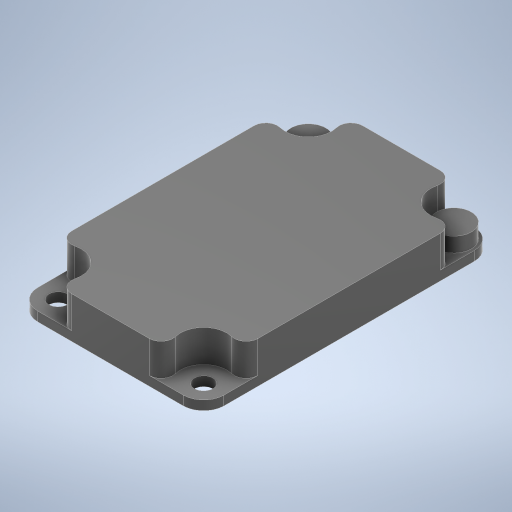
# Autodesk Inventor part: SEN0539-EN
Saved by Autodesk Inventor 2024.2 (Build 282272000, 272)
## iProperties
Created: 2024-02-11
Part Number: SEN0539-EN
Material: CFRP
Document SubType Name: Modeling
Designer: Masato Kubotera
Appearance: Smooth - Black
Surface Area: 10.415 cm^2
Volume: 0.704292 cm^3
Vendor: DFROBOT
Catalog Web Link: https://www.dfrobot.com/product-2665.html
Author: Masato Kubotera
Autodesk Inventor part; units mm, degrees
ref_plane "YZ Plane" through (0, 0, 0) normal (1, 0, 0) x (0, 1, 0)
ref_plane "XZ Plane" through (0, 0, 0) normal (0, 1, 0) x (-1, 0, 0)
ref_plane "XY Plane" through (0, 0, 0) normal (0, 0, 1) x (1, 0, 0)
sketch "Sketch1" plane through (0, 0, 0) normal (0, 0, 1) x (1, 0, 0)
  line L0 (25, 16) -> (-25, 16)
  line L1 (-25, 16) -> (-25, -16)
  line L2 (-25, -16) -> (25, -16)
  line L3 (25, -16) -> (25, 16)
  line L4 (25, 16) -> (-25, -16) construction
  line L5 (-25, 16) -> (25, -16) construction
  line L6 (0, 16) -> (0, -16) construction
  line L7 (25, 0) -> (-25, 0) construction
  line L8 (0, -16) -> (0, 16) construction
  line L9 (21.5, -12.5) -> (21.5, 12.5) construction
  circle A0 centre (-21.5, -12.5) radius 3
  circle A1 centre (-21.5, 12.5) radius 3
  arc A2 (-19.5635, -16) -> (-25, -10.5635) centre (-21.5, -12.5) ccw
  arc A3 (-25, 10.5635) -> (-19.5635, 16) centre (-21.5, 12.5) ccw
  arc A4 (25, -10.5635) -> (19.5635, -16) centre (21.5, -12.5) ccw
  arc A5 (19.5635, 16) -> (25, 10.5635) centre (21.5, 12.5) ccw
  point P0 (0, 0)
  point P1 (21.5, 0)
  point P2 (25, 10.5635)
  point P3 (19.5635, 16)
  point P4 (-19.5635, 16)
  point P5 (-25, 10.5635)
  point P6 (19.5635, -16)
  point P7 (25, -10.5635)
  dimension "d0" = 50
  dimension "d1" = 32
  dimension "d18" = 3.5
  dimension "d19" = 25
  dimension "d21" = 6
  dimension "d24" = 1
  constraints: 20 end point, 11 symmetric about line, 8 point on circle, 7 midpoint, 6 centre point, 3 coincident, 3 point on line, 2 parallel, 1 equal radius, 1 horizontal, 1 perpendicular, 1 vertical, 3 other
  measures "d0" distance of L2.end L1.end
  measures "d1" distance of L1.end L0.end
  measures "d18" distance between parallel lines of L3 L9
  measures "d19" distance of L9.start L9.end
  measures "d21" diameter of A0
  measures "d24" radial gap between concentric circles of A2 A0
extrude "Extrusion1" add sketch "Sketch1" against normal blind 1.6 contours L3 A5 L0 | A5 L3 A4 L2 A2 L1 A3 L0 | A3 L1 L0 | L3 L2 A4 | A2 L2 L1 | A0 | A1
extrude "Extrusion2" add sketch "Sketch1" along normal blind 2.5 contours A0 | A1
hole "Phi3.2" at (21.5, -12.5, 0) at (21.5, 12.5, 0) direction (0, 0, -1) diameter 3.2 end through all
fillet "R3.5" radius 3.5 4 edges at (25, -16, -0.8) (-25, -16, -0.8) (-25, 16, -0.8) (25, 16, -0.8)
extrude "Extrusion3" add sketch "Sketch1" along normal blind 5.5 contours A5 L3 A4 L2 A2 L1 A3 L0
fillet "R2" radius 2 8 edges at (19.5635, -16, 2.75) (25, -10.5635, 2.75) (25, 10.5635, 2.75) (19.5635, 16, 2.75) (-19.5635, -16, 2.75) (-25, -10.5635, 2.75) (-25, 10.5635, 2.75) (-19.5635, 16, 2.75)
equation "\"d18\" = -0.5 * d19 + 0.5 * d1"
body "Solid1"
